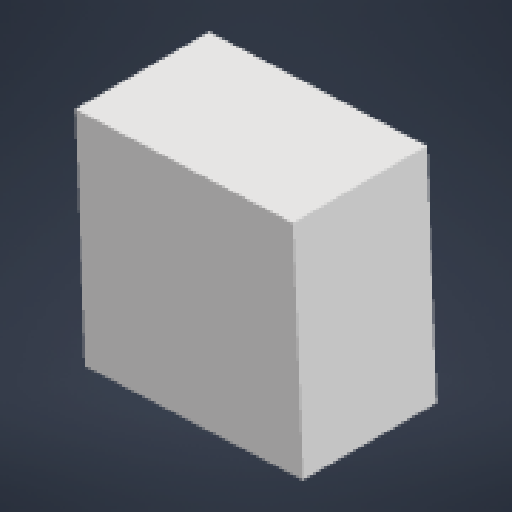
# Autodesk Inventor part: main axel
Saved by Autodesk Inventor 2026 (Build 300175050, 175E)
## iProperties
Created: 2026-04-07
Part Number: main axel
Material: Generic
Document SubType Name: Modeling
Designer: sniel
Density: 1 g/cm^3
Appearance: Default
Author: sniel
Autodesk Inventor part; units mm, degrees
ref_plane "YZ Plane" through (0, 0, 0) normal (1, 0, 0) x (0, 1, 0)
ref_plane "XZ Plane" through (0, 0, 0) normal (0, 1, 0) x (-1, 0, 0)
ref_plane "XY Plane" through (0, 0, 0) normal (0, 0, 1) x (1, 0, 0)
sketch "Sketch1" plane through (0, 0, 0) normal (0, 0, 1) x (1, 0, 0)
  line L0 (4.2481, -3.8751) -> (-3.8751, -4.2481) projected
  line L1 (3.8751, 4.2481) -> (4.2481, -3.8751) projected
  line L2 (-4.2481, 3.8751) -> (3.8751, 4.2481) projected
  line L3 (-3.8751, -4.2481) -> (-4.2481, 3.8751) projected
  arc A0 (-0.3054, 6.0062) -> (0.3054, -6.0062) centre (0, 0) ccw projected
  circle A1 centre (0, 0) radius 5.75
  point P0 (0, 0)
  constraints: 1 coincident, 3 other
extrude "Extrusion1" add sketch "Sketch1" along normal blind 3 contours L0 L3 L2 L1
sketch "Sketch2" plane through (0, 0, 3) normal (0, 0, 1) x (1, 0, 0)
  arc A0 (-0.3054, 6.0062) -> (0.3054, -6.0062) centre (0, 0) ccw
  line L0 (-3.8751, -4.2481) -> (4.2481, -3.8751) projected
  circle A1 centre (0, 0) radius 5.75
  point P0 (0, 0)
  constraints: 2 point on circle, 1 centre point, 1 coincident, 3 other
extrude "Extrusion2" add sketch "Sketch2" along normal blind 5
body "Solid1"
